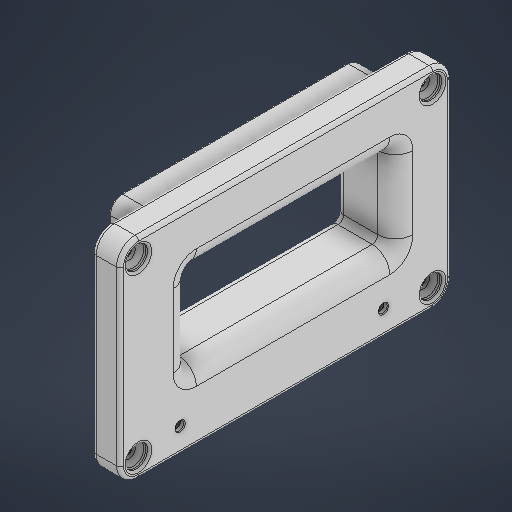
# Autodesk Inventor part: ScreenMountPlate
Saved by Autodesk Inventor 2026.2 (Build 302298010, 298A)
## iProperties
Created: 2026-03-07
Part Number: ScreenMountPlate
Material: Generic
Document SubType Name: Modeling
Designer: DanAr
Density: 1 g/cm^3
Appearance: Default
Author: DanAr
Autodesk Inventor part; units mm, degrees
ref_plane "YZ Plane" through (0, 0, 0) normal (1, 0, 0) x (0, 1, 0)
ref_plane "XZ Plane" through (0, 0, 0) normal (0, 1, 0) x (-1, 0, 0)
ref_plane "XY Plane" through (0, 0, 0) normal (0, 0, 1) x (1, 0, 0)
sketch "Sketch1" plane through (0, 0, 0) normal (1, 0, 0) x (0, 1, 0)
  line L0 (0, 0) -> (52.6, 0)
  line L1 (52.6, 0) -> (52.6, -71.4)
  line L2 (52.6, -71.4) -> (0, -71.4)
  line L3 (0, -71.4) -> (0, 0)
  line L4 (0, 0) -> (3.5, 0)
  line L5 (3.5, 0) -> (3.5, -3.5)
  line L6 (3.5, -3.5) -> (0, -3.5)
  line L7 (0, -3.5) -> (0, 0)
  circle A0 centre (3.5, -3.5) radius 2.9
  line L8 (3.5, -3.5) -> (3.5, -61.5)
  circle A1 centre (3.5, -61.5) radius 2.9
  line L9 (0, 0) -> (16, 0)
  line L10 (16, 0) -> (16, -6.5)
  line L11 (16, -6.5) -> (0, -6.5)
  line L12 (0, -6.5) -> (0, 0)
  line L13 (0, 0) -> (40, 0)
  line L14 (40, 0) -> (40, -6.5)
  line L15 (40, -6.5) -> (0, -6.5)
  line L16 (0, -6.5) -> (0, 0)
  line L17 (40, -6.5) -> (16, -6.5)
  line L18 (16, -6.5) -> (16, -64.9)
  line L19 (16, -64.9) -> (40, -64.9)
  line L20 (40, -64.9) -> (40, -6.5)
  dimension "d0" = 71.4
  dimension "d1" = 52.6
  dimension "d2" = 3.5
  dimension "d3" = 3.5
  dimension "d4" = 5.8
  dimension "d5" = 58
  dimension "d6" = 6.5
  dimension "d7" = 16
  dimension "d8" = 40
  dimension "d10" = 6.5
  dimension "d11" = 6.5
  constraints: 42 end point, 10 parallel, 5 horizontal, 5 perpendicular, 2 centre point, 2 coincident, 1 vertical
  measures "d0" distance of L0.end L1.end
  measures "d1" distance of L1.end L2.end
  measures "d2" distance of L4.end L5.end
  measures "d3" distance of L5.end L6.end
  measures "d4" diameter of A0
  measures "d5" distance of L8.start L8.end
  measures "d6" distance of L9.end L10.end
  measures "d7" distance of L10.end L11.end
  measures "d8" distance of L14.end L15.end
  measures "d10" distance between parallel lines of L2 L19
  measures "d11" distance between parallel lines of L0 L15
extrude "Extrusion1" add sketch "Sketch1" along normal blind 1 contours L0 L5 A0 L6 L3 | L0 L10 L11 L8 A0 L5 | L6 A0 L8 L11 L3 | L0 L14 L15 L10 | L11 L18 L19 L20 L14 L0 L1 L2 L3
sketch "Sketch2" plane through (1, 0, 0) normal (1, 0, 0) x (0, 0, -1)
  line L0 (0, 52.6) -> (0, 0) projected
  line L1 (71.4, 0) -> (71.4, 52.6) projected
  line L2 (0, 52.6) -> (71.4, 52.6)
  line L3 (71.4, 52.6) -> (71.4, 0)
  line L4 (71.4, 0) -> (0, 0)
  line L5 (0, 0) -> (0, 52.6)
  circle A0 centre (3.5, 3.5) radius 2.9 projected
  line L6 (3.5, 3.5) -> (67.9, 3.5)
  line L7 (67.9, 3.5) -> (67.9, 49.1)
  line L8 (67.9, 49.1) -> (3.5, 49.1)
  line L9 (3.5, 49.1) -> (3.5, 3.5)
  circle A1 centre (3.5, 3.5) radius 3.5
  circle A2 centre (3.5, 49.1) radius 3.5
  circle A3 centre (67.9, 49.1) radius 3.5
  circle A4 centre (67.9, 3.5) radius 3.5
  line L10 (6.5, 40) -> (64.9, 40) projected
  line L11 (64.9, 40) -> (64.9, 16) projected
  line L12 (6.5, 40) -> (64.9, 40)
  line L13 (64.9, 40) -> (64.9, 16)
  line L14 (64.9, 16) -> (6.5, 16)
  line L15 (6.5, 16) -> (6.5, 40)
  point P0 (0, 3.5)
  point P1 (3.5, 0)
  point P2 (67.9, 0)
  point P3 (71.4, 3.5)
  point P4 (71.4, 49.1)
  point P5 (67.9, 52.6)
  point P6 (3.5, 52.6)
  point P7 (0, 49.1)
  dimension "d14" = 3.5
  dimension "d15" = 3.5
  constraints: 24 end point, 6 parallel, 4 centre point, 4 coincident, 4 tangent, 3 horizontal, 3 perpendicular
  measures "d14" distance between parallel lines of L2 L8
  measures "d15" distance between parallel lines of L1 L7
extrude "Extrusion2" add sketch "Sketch2" against normal blind 9 contours A2 L9 A1 L0 | A2 L8 L9 | L2 A3 L8 A2 | A1 L9 A0 L6 | A2 L8 A3 L7 A4 L6 A1 L9 | L9 L8 A2 | A3 L7 L8 | A1 L6 A0 L9 | A1 L6 A4 L4 | L1 A4 L7 A3 | L8 L7 A3 | L9 L6 A0 | A0 L6 L9 | A4 L6 L7 | A4 L7 L6
fillet "Fillet1" radius 0.4 8 edges at (-8, 52.6, -35.7) (-8, 51.5749, -1.0251) (-8, 26.3, 0) (-8, 1.0251, -1.0251) (-8, 0, -35.7) (-8, 1.0251, -70.3749) (-8, 26.3, -71.4) (-8, 51.5749, -70.3749)
fillet "Fillet2" radius 1.6 4 edges at (-3.5, 16, -64.9) (-3.5, 40, -64.9) (-3.5, 40, -6.5) (-3.5, 16, -6.5)
fillet "Fillet3" radius 2 7 edges at (-8, 40, -35.7) (-8, 39.5314, -64.4314) (-8, 28, -64.9) (-8, 16.4686, -64.4314) (-8, 16, -35.7) (-8, 28, -6.5) (-8, 39.5314, -6.9686)
sketch "Sketch3" plane through (1, 3.5, -3.5) normal (1, 0, 0) x (0, 0, 1)
  circle A0 centre (-58, 0) radius 2.9 projected
  circle A1 centre (-58, 0) radius 2.9
  circle A2 centre (0, 0) radius 2.9 projected
  circle A3 centre (0, 0) radius 2.9
  point P0 (3.5, 3.5)
  constraints: 2 centre point, 2 coincident
extrude "Extrusion3" cut sketch "Sketch3" against normal blind 9
fillet "Fillet4" radius 0.2 2 edges at (-8, 3.5, -64.4) (-8, 3.5, -6.4)
sketch "Sketch5" plane through (1, 0, 0) normal (1, 0, 0) x (0, 0, -1)
  line L0 (6.5, 38.4) -> (6.5, 17.6) projected
  arc A0 (8.1, 40) -> (6.5, 38.4) centre (8.1, 38.4) ccw projected
  line L1 (6.5, 38.4) -> (8.1, 38.4)
  line L2 (8.1, 38.4) -> (8.1, 40)
  line L3 (8.1, 40) -> (6.5, 40)
  line L4 (6.5, 40) -> (6.5, 38.4)
  line L5 (6.5, 40) -> (64.9, 40)
  line L6 (64.9, 40) -> (64.9, 16)
  line L7 (64.9, 16) -> (6.5, 16)
  line L8 (6.5, 16) -> (6.5, 40)
  line L9 (0, 0) -> (71.4, 0) projected
  line L10 (35.7, 0) -> (35.7, 52.6)
  line L11 (3.5, 52.6) -> (67.9, 52.6) projected
  line L12 (35.7, 26.3) -> (33.55, 26.3)
  line L13 (75.5, 1.75) -> (-8.4, 1.75)
  line L14 (-8.4, 1.75) -> (-8.4, 50.85)
  line L15 (-8.4, 50.85) -> (75.5, 50.85)
  line L16 (75.5, 50.85) -> (75.5, 1.75)
  line L17 (75.5, 1.75) -> (-8.4, 50.85) construction
  line L18 (-8.4, 1.75) -> (75.5, 50.85) construction
  line L19 (71.55, -0.15) -> (-0.15, -0.15)
  line L20 (-0.15, -0.15) -> (-0.15, 52.75)
  line L21 (-0.15, 52.75) -> (71.55, 52.75)
  line L22 (71.55, 52.75) -> (71.55, -0.15)
  line L23 (71.55, -0.15) -> (-0.15, 52.75) construction
  line L24 (-0.15, -0.15) -> (71.55, 52.75) construction
  circle A1 centre (-8.4, 50.85) radius 2.25
  circle A2 centre (75.5, 50.85) radius 2.25
  circle A3 centre (-8.4, 1.75) radius 2.25
  circle A4 centre (75.5, 1.75) radius 2.25
  line L25 (80.75, -3.5) -> (-13.65, -3.5)
  line L26 (-13.65, -3.5) -> (-13.65, 56.1)
  line L27 (-13.65, 56.1) -> (80.75, 56.1)
  line L28 (80.75, 56.1) -> (80.75, -3.5)
  line L29 (80.75, -3.5) -> (-13.65, 56.1) construction
  line L30 (-13.65, -3.5) -> (80.75, 56.1) construction
  circle A5 centre (8.1, 38.4) radius 1.6
  arc A6 (64.9, 38.4) -> (63.3, 40) centre (63.3, 38.4) ccw projected
  line L31 (64.9, 38.4) -> (66.9, 38.4) projected
  circle A7 centre (63.3, 38.4) radius 1.6
  arc A8 (63.3, 16) -> (64.9, 17.6) centre (63.3, 17.6) ccw projected
  line L32 (64.9, 17.6) -> (64.9, 38.4) projected
  circle A9 centre (63.3, 17.6) radius 1.6
  arc A10 (6.5, 17.6) -> (8.1, 16) centre (8.1, 17.6) ccw projected
  circle A11 centre (8.1, 17.6) radius 1.6
  circle A12 centre (3.5, 3.5) radius 2.9 projected
  circle A13 centre (3.5, 3.5) radius 2.9
  circle A14 centre (61.5, 3.5) radius 3.1 projected
  circle A15 centre (61.5, 3.5) radius 2.9
  point P0 (61.5, 0.4)
  dimension "d24" = 2.15
  dimension "d25" = 83.9
  dimension "d26" = 71.7
  dimension "d27" = 52.9
  dimension "d28" = 8.25
  dimension "d31" = 3.95
  dimension "d32" = 49.1
  dimension "d33" = 4.5
  dimension "d34" = 5.25
  dimension "d35" = 5.25
  dimension "d37" = 5.8
  dimension "d38" = 5.8
  constraints: 56 end point, 10 coincident, 10 parallel, 9 midpoint, 6 centre point, 6 horizontal, 5 perpendicular, 3 vertical alignment, 2 horizontal alignment, 8 other
  measures "d24" distance of L12.start L12.end
  measures "d25" distance of L14.end L15.end
  measures "d26" distance of L20.end L21.end
  measures "d27" distance of L19.end L20.end
  measures "d28" distance between parallel lines of L14 L20
  measures "d31" distance between parallel lines of L22 L16
  measures "d32" distance of L15.end L13.start
  measures "d33" diameter of A1
  measures "d34" distance from line of L27 A1.centre
  measures "d35" distance from line of L26 A1.centre
  measures "d37" diameter of A15
  measures "d38" diameter of A13
extrude "Extrusion4" add sketch "Sketch5" along normal blind 4 contours L4 L3 A0 | L0 L8 L7 L10 L13 A12 L20 L15 L5 L3 L4 | A10 L7 L8 | L10 L15 L22 L13 A14 L7 L6 L5 | L5 L6 A6 | L15 L20 L21 L22 | A8 L6 L7 | L13 A14 L22 L19 L20 A12 | L20 L13 A3 L14 A1 L15 | L15 A2 L16 A4 L13 L22 | A14 L13 A15 | L13 A15 A14 | L25 L26 L27 L28
fillet "Fillet5" radius 5.25 4 edges at (3, 56.1, 13.65) (3, 56.1, -80.75) (3, -3.5, -80.75) (3, -3.5, 13.65)
sketch "Sketch6" plane through (5, 0, 0) normal (1, 0, 0) x (0, 0, -1)
  arc A0 (-8.4, 56.1) -> (-13.65, 50.85) centre (-8.4, 50.85) ccw projected
  line L0 (-8.4, 56.1) -> (-13.65, 56.1)
  line L1 (-13.65, 56.1) -> (-13.65, 50.85)
  line L2 (-13.65, 50.85) -> (-8.4, 50.85)
  line L3 (-8.4, 50.85) -> (-8.4, 56.1)
  line L4 (-13.65, 56.1) -> (80.75, 56.1)
  line L5 (80.75, 56.1) -> (80.75, -3.5)
  line L6 (80.75, -3.5) -> (-13.65, -3.5)
  line L7 (-13.65, -3.5) -> (-13.65, 56.1)
  circle A1 centre (-8.4, 50.85) radius 2.25 projected
  circle A2 centre (-8.4, 50.85) radius 1.5
  circle A3 centre (-8.4, 1.75) radius 2.25 projected
  circle A4 centre (-8.4, 1.75) radius 1.5
  circle A5 centre (75.5, 1.75) radius 2.25 projected
  circle A6 centre (75.5, 1.75) radius 1.5
  circle A7 centre (75.5, 50.85) radius 2.25 projected
  circle A8 centre (75.5, 50.85) radius 1.5
  circle A9 centre (3.5, 3.5) radius 2.9 projected
  circle A10 centre (3.5, 3.5) radius 2.9
  circle A11 centre (61.5, 3.5) radius 2.9 projected
  circle A12 centre (61.5, 3.5) radius 2.9
  arc A13 (8.1, 40) -> (6.5, 38.4) centre (8.1, 38.4) ccw projected
  circle A14 centre (8.1, 38.4) radius 1.6
  arc A15 (64.9, 38.4) -> (63.3, 40) centre (63.3, 38.4) ccw projected
  circle A16 centre (63.3, 38.4) radius 1.6
  arc A17 (63.3, 16) -> (64.9, 17.6) centre (63.3, 17.6) ccw projected
  line L8 (64.9, 38.4) -> (64.9, 17.6) projected
  circle A18 centre (63.3, 17.6) radius 1.6
  arc A19 (6.5, 17.6) -> (8.1, 16) centre (8.1, 17.6) ccw projected
  circle A20 centre (8.1, 17.6) radius 1.6
  line L9 (6.5, 38.4) -> (64.9, 38.4)
  line L10 (64.9, 38.4) -> (64.9, 17.6)
  line L11 (64.9, 17.6) -> (6.5, 17.6)
  line L12 (6.5, 17.6) -> (6.5, 38.4)
  line L13 (63.3, 16) -> (8.1, 16)
  line L14 (8.1, 16) -> (8.1, 40)
  line L15 (8.1, 40) -> (63.3, 40)
  line L16 (63.3, 40) -> (63.3, 16)
  circle A21 centre (-8.4, 50.85) radius 5.25
  circle A22 centre (75.5, 50.85) radius 5.25
  circle A23 centre (75.5, 1.75) radius 5.25
  circle A24 centre (-8.4, 1.75) radius 5.25
  point P0 (0, 0)
  point P1 (-13.65, 50.85)
  point P2 (-13.65, 1.75)
  point P3 (-8.4, -3.5)
  point P4 (75.5, -3.5)
  point P5 (80.75, 1.75)
  point P6 (80.75, 50.85)
  point P7 (75.5, 56.1)
  point P8 (63.3, 40)
  point P9 (8.1, 16)
  point P10 (6.5, 17.6)
  dimension "d42" = 3
  constraints: 32 end point, 14 coincident, 9 centre point, 8 parallel, 4 horizontal, 4 perpendicular, 4 vertical alignment, 3 tangent, 1 horizontal alignment, 10 other
  measures "d42" diameter of A2
extrude "Extrusion5" add sketch "Sketch6" along normal blind 2.5 contours L3 A1 L2 A0 | A21 L2 A1 L3 | L4 A22 L5 A23 L6 A24 L7 A21 | A1 L2 A2 L3 | L3 A2 L2 A1 | A22 | A24 | A23 | A3 | A5 | A7
chamfer "Chamfer1" distance 1.7 angle 45 4 edges at (7.5, 50.85, 9.9) (7.5, 50.85, -74) (7.5, 1.75, -74) (7.5, 1.75, 9.9)
fillet "Fillet6" radius 1 4 edges at (5.8, 1.75, -74) (5.8, 50.85, -74) (5.8, 50.85, 9.9) (5.8, 1.75, 9.9)
sketch "Sketch7" plane through (7.5, 0, 0) normal (1, 0, 0) x (0, 0, -1)
  circle A0 centre (-8.4, 50.85) radius 3.2 projected
  circle A1 centre (-8.4, 50.85) radius 3.2
  circle A2 centre (75.5, 50.85) radius 3.2 projected
  circle A3 centre (75.5, 50.85) radius 3.2
  circle A4 centre (75.5, 1.75) radius 3.2 projected
  circle A5 centre (75.5, 1.75) radius 3.2
  circle A6 centre (-8.4, 1.75) radius 3.2 projected
  circle A7 centre (-8.4, 1.75) radius 3.2
  circle A8 centre (3.5, 3.5) radius 2.9 projected
  circle A9 centre (3.5, 3.5) radius 1.25
  circle A10 centre (61.5, 3.5) radius 2.9 projected
  circle A11 centre (61.5, 3.5) radius 1.25
  arc A12 (-8.4, 56.1) -> (-13.65, 50.85) centre (-8.4, 50.85) ccw projected
  circle A13 centre (-8.4, 50.85) radius 5.25
  arc A14 (80.75, 50.85) -> (75.5, 56.1) centre (75.5, 50.85) ccw projected
  circle A15 centre (75.5, 50.85) radius 5.25
  arc A16 (75.5, -3.5) -> (80.75, 1.75) centre (75.5, 1.75) ccw projected
  circle A17 centre (75.5, 1.75) radius 5.25
  circle A18 centre (-8.4, 1.75) radius 1.5 projected
  arc A19 (-13.65, 1.75) -> (-8.4, -3.5) centre (-8.4, 1.75) ccw projected
  circle A20 centre (-8.4, 1.75) radius 5.25
  line L0 (-8.4, -3.5) -> (-13.65, -3.5)
  line L1 (-13.65, -3.5) -> (-13.65, 1.75)
  line L2 (-13.65, -3.5) -> (80.75, -3.5)
  line L3 (80.75, -3.5) -> (80.75, 56.1)
  line L4 (80.75, 56.1) -> (-13.65, 56.1)
  line L5 (-13.65, 56.1) -> (-13.65, -3.5)
  arc A21 (8.1, 40) -> (6.5, 38.4) centre (8.1, 38.4) ccw projected
  circle A22 centre (8.1, 38.4) radius 1.6
  arc A23 (6.5, 17.6) -> (8.1, 16) centre (8.1, 17.6) ccw projected
  circle A24 centre (8.1, 17.6) radius 1.6
  arc A25 (63.3, 16) -> (64.9, 17.6) centre (63.3, 17.6) ccw projected
  circle A26 centre (63.3, 17.6) radius 1.6
  arc A27 (64.9, 38.4) -> (63.3, 40) centre (63.3, 38.4) ccw projected
  circle A28 centre (63.3, 38.4) radius 1.6
  line L6 (63.3, 40) -> (8.1, 40) projected
  line L7 (8.1, 40) -> (63.3, 40)
  line L8 (63.3, 40) -> (63.3, 16)
  line L9 (63.3, 16) -> (8.1, 16)
  line L10 (8.1, 16) -> (8.1, 40)
  line L11 (6.5, 38.4) -> (4.5, 38.4) projected
  line L12 (64.9, 17.6) -> (6.5, 17.6)
  line L13 (6.5, 17.6) -> (6.5, 38.4)
  line L14 (6.5, 38.4) -> (64.9, 38.4)
  line L15 (64.9, 38.4) -> (64.9, 17.6)
  point P0 (0, 0)
  point P1 (-13.65, 50.85)
  point P2 (-13.65, 1.75)
  point P3 (-8.4, -3.5)
  point P4 (80.75, 1.75)
  point P5 (8.1, 16)
  point P6 (6.5, 17.6)
  dimension "d49" = 2.5
  constraints: 28 end point, 14 coincident, 7 vertical alignment, 6 centre point, 6 parallel, 4 horizontal, 4 perpendicular, 1 horizontal alignment, 16 other
  measures "d49" diameter of A9
extrude "Extrusion6" add sketch "Sketch7" along normal blind 1.3 contours A8 | A10 | A13 A12 | L4 A15 L3 A17 L2 A20 L5 A13 | A14 A15 | A20 A19 | A16 A17
fillet "Fillet7" radius 5 8 edges at (8.8, 16, -35.7) (8.8, 16.4686, -6.9686) (8.8, 28, -6.5) (8.8, 39.5314, -6.9686) (8.8, 40, -35.7) (8.8, 39.5314, -64.4314) (8.8, 28, -64.9) (8.8, 16.4686, -64.4314)
fillet "Fillet8" radius 0.6 4 edges at (7.5, 1.75, -72.3) (7.5, 50.85, -72.3) (7.5, 50.85, 11.6) (7.5, 1.75, 11.6)
fillet "Fillet9" radius 0.6 4 edges at (8.8, 50.85, 11.6) (8.8, 50.85, -72.3) (8.8, 1.75, -72.3) (8.8, 1.75, 11.6)
chamfer "Chamfer2" distance 0.2 angle 45 4 edges at (8.8, 3.5, -2.25) (7.5, 3.5, -2.25) (8.8, 3.5, -60.25) (7.5, 3.5, -60.25)
fillet "Fillet10" radius 1 16 edges at (8.8, 56.1, -33.55) (8.8, 54.5623, 12.1123) (8.8, 26.3, 13.65) (8.8, -1.9623, 12.1123) (8.8, -3.5, -33.55) (8.8, -1.9623, -79.2123) (8.8, 26.3, -80.75) (8.8, 54.5623, -79.2123) (1, 26.3, 13.65) (1, -1.9623, 12.1123) (1, -3.5, -33.55) (1, -1.9623, -79.2123) (1, 26.3, -80.75) (1, 54.5623, -79.2123) (1, 56.1, -33.55) (1, 54.5623, 12.1123)
fillet "Fillet11" radius 1 4 edges at (1, 50.85, 10.65) (1, 1.75, 10.65) (1, 50.85, -73.25) (1, 1.75, -73.25)
fillet "Fillet12" radius 0.5 4 edges at (0, 51.5749, -70.3749) (0, 51.5749, -1.0251) (0, 1.0251, -70.3749) (0, 1.0251, -1.0251)
fillet "Fillet13" radius 0.3 4 edges at (0.5, 52.6, 0) (0.5, 52.6, -71.4) (0.5, 0, 0) (0.5, 0, -71.4)
fillet "Fillet14" radius 0.2 20 edges at (0, 0.9318, -71.4) (-0.1605, 2.5262, -71.4) (0, 0.0879, -71.3121) (0, 0, -70.4682) (-0.1605, 0, -68.8738) (0, 52.6, -70.4682) (0, 52.5121, -71.3121) (0, 51.6682, -71.4) (-0.1605, 50.0738, -71.4) (-0.1605, 52.6, -68.8738) (0, 52.5121, -0.0879) (0, 51.6682, 0) (-0.1359, 50.161, 0) (-0.1605, 52.6, -2.5262) (0, 52.6, -0.9318) (0, 0.0879, -0.0879) (0, 0, -0.9318) (-0.1605, 0, -2.5262) (-0.1605, 2.5262, 0) (0, 0.9318, 0)
chamfer "Chamfer3" distance 0.2 angle 45 4 edges at (5, 1.75, 9.9) (5, 1.75, -74) (5, 50.85, -74) (5, 50.85, 9.9)
body "Solid1"
